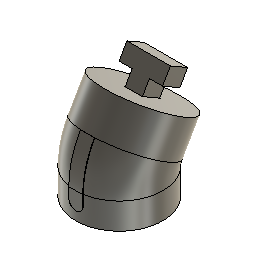
MakeupMirrorMount (Autodesk Fusion 360 design; units mm, degrees)
part number: 2026-05-30-17-06-30-521
Autodesk Fusion 360 part; units mm, degrees
sketch "Sketch1" plane through (0, 0, 0) normal (0, 0, 1) x (1, 0, 0)
  line L0 (0, 0) -> (17.6777, 17.6777)
  line L1 (0, 0) -> (50, 0) construction
  line L2 (0, 0) -> (-17.6777, 17.6777)
  arc A0 (-17.6777, 17.6777) -> (17.6777, 17.6777) centre (0, 0) ccw
  arc A1 (-11.3137, 11.3137) -> (11.3137, 11.3137) centre (0, 0) ccw
  dimension "d1" = 32
  dimension "d2" = 50
  dimension "d6" = 45
  constraint coincident L0.start L1.start
  constraint horizontal L1
  constraint coincident L0 A1.end
  constraint coincident L2 A1.start
  measures "d1" diameter of A1
  measures "d2" diameter of A0
  measures "d6" angle of L0 L1
extrude "Extrude2" add sketch "Sketch1" along normal blind 15 contours L0 L2 A0 A1 makes body 1
ref_plane "WorkPlane1" through (0, -25, 4.7618) normal (0, -1, 0) x (-1, 0, 0)
sketch "Sketch2" plane through (0, -25, 0) normal (0, -1, 0) x (-1, 0, 0)
  line L0 (4, -15) -> (-4, -15)
  line L1 (-4, -15) -> (-4, -9)
  line L2 (4, -9) -> (4, -15)
  line L3 (4, -15) -> (-4, -5) construction
  line L4 (-4, -15) -> (4, -5) construction
  arc A0 (4, -9) -> (0, -5) centre (0, -9) ccw
  arc A1 (0, -5) -> (-4, -9) centre (0, -9) ccw
  point P0 (0, -10)
  dimension "d11" = 8
  dimension "d12" = 10
  dimension "d14" = 4
  dimension "d15" = 4
  constraint horizontal L0
  constraint perpendicular L0 L1
  constraint parallel L1 L2
  constraint coincident L3 P0
  constraint coincident L4 P0
  constraint coincident L4.end L2
  constraint tangent L2 A0
  constraint coincident L3.end L1
  constraint tangent L1 A1
  constraint coincident A0.end A1.start
  measures "d11" distance of L3.end L4.end
  measures "d12" distance of L0.end L3.end
  measures "d14" radius of A0
  measures "d15" radius of A1
extrude "Extrude3" add sketch "Sketch2" against normal blind 50 bodies 1
revolve "Revolve1" add 1 faces at (-1.3333, 11.5027, 15) angle 30 about axis through (-4, 25, 15) along (-1, 0, 0) on bodies 1 bodies 1
sketch "Sketch3" plane through (0, 12.7452, 22.0753) normal (0, 0.5, 0.866025) x (-1, 0, 0)
  arc A0 (-4, 35.5273) -> (-17.6777, -6.8283) centre (0, 10.8494) ccw
  line L0 (-17.6777, -6.8283) -> (-11.3137, -0.4643)
  arc A1 (-4, 26.3413) -> (-11.3137, -0.4643) centre (0, 10.8494) ccw
  line L1 (-4, 26.3413) -> (-4, -14.1506)
  line L2 (-4, -14.1506) -> (4, -14.1506)
  line L3 (4, -14.1506) -> (4, 26.3413)
  arc A2 (11.3137, -0.4643) -> (4, 26.3413) centre (0, 10.8494) ccw
  line L4 (11.3137, -0.4643) -> (17.6777, -6.8283)
  arc A3 (17.6777, -6.8283) -> (4, 35.5273) centre (0, 10.8494) ccw
  line L5 (4, 35.5273) -> (4, 35.8494)
  line L6 (4, 35.8494) -> (-4, 35.8494)
  line L7 (-4, 35.8494) -> (-4, 35.5273)
  circle A4 centre (0, 10.8494) radius 25
  constraint concentric A0 A4
extrude "Extrude4" add sketch "Sketch3" along normal blind 20 contours A0 L0 A1 L1 L3 A2 L4 A3 A4 | L0 A1 L1 A4 | L3 A2 L4 A4 bodies 1
sketch "Sketch4" plane through (0, 22.7452, 39.3958) normal (0, 0.5, 0.866025) x (-1, 0, 0)
  circle A0 centre (0, 10.8494) radius 25
  line L0 (5.1, 16.8994) -> (-5.1, 16.8994)
  line L1 (-5.1, 16.8994) -> (-5.1, 4.7994)
  line L2 (-5.1, 4.7994) -> (5.1, 4.7994)
  line L3 (5.1, 4.7994) -> (5.1, 16.8994)
  line L4 (5.1, 16.8994) -> (-5.1, 4.7994) construction
  line L5 (-5.1, 16.8994) -> (5.1, 4.7994) construction
  point P0 (0, 10.8494)
  dimension "d21" = 10.2
  dimension "d22" = 12.1
  constraint horizontal L0
  constraint perpendicular L0 L1
  constraint parallel L0 L2
  constraint parallel L1 L3
  constraint coincident L4 P0
  constraint coincident L5 P0
  constraint coincident P0 A0.centre
  measures "d21" distance of L1.end L2.end
  measures "d22" distance of L0.end L1.end
extrude "Extrude5" cut sketch "Sketch4" against normal blind 19 contours L0 L1 L2 L3 bodies 1
sketch "Sketch8" plane through (0, 13.2452, 22.9413) normal (0, 0.5, 0.866025) x (-1, 0, 0)
  line L0 (5.1, 4.7994) -> (5.1, 16.8994)
  line L1 (5.1, 16.8994) -> (-5.1, 16.8994)
  line L2 (-5.1, 16.8994) -> (-5.1, 4.7994)
  line L3 (-5.1, 4.7994) -> (5.1, 4.7994)
  line L4 (-5.1, 4.7994) -> (5.1, 4.7994)
  line L5 (5.1, 4.7994) -> (5.1, 16.8994)
  line L6 (5.1, 16.8994) -> (-5.1, 16.8994)
  line L7 (-5.1, 16.8994) -> (-5.1, 4.7994)
  constraint horizontal L4
  constraint vertical L5
  constraint horizontal L6
  constraint vertical L7
  constraint coincident L0.end L1.start
  constraint coincident L2.end L3.start
extrude "Extrude8" add sketch "Sketch8" along normal blind 27 separate body makes body 2
sketch "Sketch10" plane through (0, 26.7452, 46.324) normal (0, 0.5, 0.866025) x (-1, 0, 0)
  line L0 (-5.1, 16.8994) -> (-5.1, 4.7994)
  line L1 (-5.1, 4.7994) -> (5.1, 4.7994)
  line L2 (5.1, 4.7994) -> (5.1, 16.8994)
  line L3 (5.1, 16.8994) -> (-5.1, 16.8994)
  line L4 (0, 4.7994) -> (0, 16.8994)
  line L5 (0, 16.8994) -> (-12.5, 16.8994)
  line L6 (-12.5, 16.8994) -> (0, 16.8994)
  line L7 (0, 16.8994) -> (0, 4.7994)
  line L8 (0, 4.7994) -> (-12.5, 4.7994)
  line L9 (-12.5, 4.7994) -> (-12.5, 16.8994)
  line L10 (0, 16.8994) -> (12.5, 16.8994)
  line L11 (12.5, 4.7994) -> (12.5, 16.8994)
  line L12 (0, 4.7994) -> (12.5, 4.7994)
  line L13 (0, 16.8994) -> (0, 4.7994)
  dimension "d39" = 12.5
  constraint midpoint L1 L4.start
  constraint midpoint L3 L4.end
  constraint perpendicular L4 L5
  constraint horizontal L6
  constraint vertical L7
  constraint horizontal L8
  constraint vertical L9
  constraint symmetric L4.start L7 L8.start
  constraint symmetric L4.end L7 L5.start
  constraint symmetric L5.end L7 L10.end
  constraint symmetric L8.end L7 L11.start
  measures "d39" distance of L4.end L5.end
extrude "Extrude9" add sketch "Sketch10" along normal blind 9 bodies 2
move_face "OffsetFaces1" offset -0.1 2 faces at (-1.7, 3.1099, 39.1853) (1.7, 18.0888, 40.9295) on bodies 2
move_face "OffsetFaces2" offset -0.15 2 faces at (5.1, 10.067, 35.1686) (-5.1, 11.1317, 44.9461) on bodies 2
move_face "OffsetFaces3" offset -0.2 2 faces at (1.65, 13.5022, 33.1853) (-1.65, 3.1965, 39.1353) on bodies 2
equation "d33 = 19 mm + 8 mm"
equation "d39 = ( 25 / 2 ) * 1 mm"
